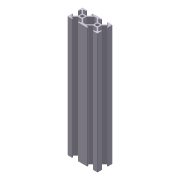
# Autodesk Inventor part: 8020-25-Double
Saved by Autodesk Inventor 2014 (Build 180170000, 170)
## iProperties
Created: 2014-08-06
Part Number: 8020-25-Double
Material: Generic
Document SubType Name: Modeling
Designer: Peele
Density: 1 g/cm^3
Appearance: Default
Author: Peele
Autodesk Inventor part; units mm, degrees
ref_plane "YZ Plane" through (0, 0, 0) normal (1, 0, 0) x (0, 1, 0)
ref_plane "XZ Plane" through (0, 0, 0) normal (0, 1, 0) x (-1, 0, 0)
ref_plane "XY Plane" through (0, 0, 0) normal (0, 0, 1) x (1, 0, 0)
sketch "Sketch1" plane through (0, 0, 0) normal (0, 0, 1) x (1, 0, 0)
  line L0 (-4.38, -4.38) -> (4.38, -4.38)
  line L1 (4.38, -4.38) -> (4.38, 4.38)
  line L2 (4.38, 4.38) -> (-4.38, 4.38)
  line L3 (-4.38, 4.38) -> (-4.38, -4.38)
  line L4 (-4.38, -4.38) -> (4.38, 4.38) construction
  line L5 (4.38, -4.38) -> (-4.38, 4.38) construction
  circle A0 centre (0, 0) radius 2.5
  dimension "d0" = 8.76
  dimension "d1" = 5
  constraints: 12 end point, 2 midpoint, 2 parallel, 2 perpendicular, 1 centre point, 1 coincident, 1 horizontal
  measures "d0" distance of L1.end L2.end
  measures "d1" diameter of A0
extrude "Extrusion1" add sketch "Sketch1" along normal mid plane 200
sketch "Sketch2" plane through (0, 0, 0) normal (0, 0, 1) x (1, 0, 0)
  line L0 (-4.38, 2.8668) -> (-10.36, 8.8468)
  line L1 (-10.36, 8.8468) -> (-10.36, 4.4)
  line L2 (-10.36, 4.4) -> (-12.5, 4.4)
  line L3 (-12.5, 4.4) -> (-12.5, 12.5)
  line L4 (-12.5, 12.5) -> (-4.4, 12.5)
  line L5 (-4.4, 12.5) -> (-4.4, 10.36)
  line L6 (-4.4, 10.36) -> (-8.8468, 10.36)
  line L7 (-8.8468, 10.36) -> (-2.8668, 4.38)
  line L8 (-2.8668, 4.38) -> (-4.38, 2.8668)
  line L9 (-4.38, 4.38) -> (4.38, 4.38) projected
  line L10 (-4.38, -4.38) -> (-4.38, 4.38) projected
  point P0 (0, 0)
  dimension "d4" = 12.5
  dimension "d5" = 2.14
  dimension "d6" = 8.1
  dimension "d7" = 2.14
  constraints: 18 end point, 6 perpendicular, 4 equal length, 2 point on line, 1 parallel, 1 vertical
  measures "d4" distance from line of point (0, 0) L4
  measures "d5" distance between parallel lines of L4 L6
  measures "d6" distance of L3.end L4.end
  measures "d7" distance between parallel lines of L0 L7
extrude "Extrusion2" add sketch "Sketch2" along normal up to surface (200 mm away) from surface at -100 contours L0 L1 L2 L3 L4 L5 L6 L7 L9 L10
pattern_circular "Circular Pattern1" count 4 over 360 about axis through (0, 0, 0) along (0, 0, 1) of "Extrusion2"
mirror "Mirror1" about plane through (12.5, 4.4, 0) normal (1, 0, 0) of "Extrusion2", "Extrusion1", "Circular Pattern1"
sketch "Sketch3" plane through (0, 0, 100) normal (0, 0, 1) x (1, 0, 0)
  line L0 (14.64, 4.4) -> (10.36, 4.4)
  line L1 (10.36, 4.4) -> (10.36, 9.2296)
  line L2 (10.36, 9.2296) -> (14.64, 9.2296)
  line L3 (14.64, 9.2296) -> (14.64, 4.4)
  line L4 (14.64, -4.4) -> (10.36, -4.4)
  line L5 (10.36, -4.4) -> (10.36, -8.8468)
  line L6 (10.36, -8.8468) -> (14.64, -8.8468)
  line L7 (14.64, -8.8468) -> (14.64, -4.4)
  constraints: 16 end point, 4 parallel, 2 horizontal, 2 perpendicular
extrude "Extrusion3" cut sketch "Sketch3" against normal up to next
fillet "Fillet4" radius 1 28 edges at (-10.36, 4.4, 0) (-10.36, -4.4, 0) (-12.5, -4.4, 0) (-12.5, 4.4, 0) (-12.5, 12.5, 0) (-4.4, 12.5, 0) (-4.4, 10.36, 0) (-4.4, -10.36, 0) (-4.4, -12.5, 0) (-12.5, -12.5, 0) (29.4, -10.36, 0) (29.4, -12.5, 0) (29.4, 10.36, 0) (29.4, 12.5, 0) (37.5, -4.4, 0) (35.36, -4.4, 0) (37.5, 12.5, 0) (37.5, -12.5, 0) (37.5, 4.4, 0) (35.36, 4.4, 0) (20.6, 10.36, 0) (20.6, 12.5, 0) (20.6, -12.5, 0) (20.6, -10.36, 0) (4.4, -12.5, 0) (4.4, -10.36, 0) (4.4, 10.36, 0) (4.4, 12.5, 0)
fillet "Fillet5" radius 0.75 16 edges at (-8.8468, -10.36, 0) (-10.36, -8.8468, 0) (8.8468, -10.36, 0) (10.36, -8.8468, 0) (14.64, -8.8468, 0) (16.1532, -10.36, 0) (33.8468, -10.36, 0) (35.36, -8.8468, 0) (33.8468, 10.36, 0) (8.8468, 10.36, 0) (35.36, 8.8468, 0) (16.1532, 10.36, 0) (14.64, 8.8468, 0) (10.36, 8.8468, 0) (-8.8468, 10.36, 0) (-10.36, 8.8468, 0)
fillet "Fillet6" radius 0.75 18 edges at (-4.38, -2.8668, 0) (-4.38, 2.8668, 0) (2.8668, 4.38, 0) (-2.8668, 4.38, 0) (-2.8668, -4.38, 0) (2.8668, -4.38, 0) (4.38, -2.8668, 0) (4.38, 2.8668, 0) (29.38, 2.8668, 0) (29.38, -2.8668, 0) (27.8668, 4.38, 0) (22.1332, 4.38, 0) (20.62, 2.8668, 0) (20.62, -2.8668, 0) (27.8668, -4.38, 0) (22.1332, -4.38, 0) (14.64, 9.2296, 0) (10.36, 9.2296, 0)
fillet "Fillet7" radius 0.75 222 edges at (-12.2071, -12.2071, 100) (-12.5, -8.45, 100) (-12.2071, -4.6929, 100) (-11.43, -4.4, 100) (-10.6529, -4.6929, 100) (-10.36, -6.2181, 100) (-9.897, -7.729, 100) (-6.8397, -5.3265, 100) (-4.4371, -2.8431, 100) (-4.38, 0, 100) (-4.4371, 2.8431, 100) (-6.8397, 5.3265, 100) (-9.897, 7.729, 100) (-10.36, 6.2181, 100) (-10.6529, 4.6929, 100) (-11.43, 4.4, 100) (-12.2071, 4.6929, 100) (-12.5, 8.45, 100) (-12.2071, 12.2071, 100) (-8.45, 12.5, 100) (-4.6929, 12.2071, 100) (-4.4, 11.43, 100) (-4.6929, 10.6529, 100) (-6.2181, 10.36, 100) (-7.729, 9.897, 100) (-5.3265, 6.8397, 100) (-2.8431, 4.4371, 100) (0, 4.38, 100) (2.8431, 4.4371, 100) (5.3265, 6.8397, 100) (7.729, 9.897, 100) (6.2181, 10.36, 100) (4.6929, 10.6529, 100) (4.4, 11.43, 100) (4.6929, 12.2071, 100) (12.5, 12.5, 100) (20.3071, 12.2071, 100) (20.6, 11.43, 100) (20.3071, 10.6529, 100) (18.7819, 10.36, 100) (17.271, 9.897, 100) (19.6735, 6.8397, 100) (22.1569, 4.4371, 100) (25, 4.38, 100) (27.8431, 4.4371, 100) (30.3265, 6.8397, 100) (32.729, 9.897, 100) (31.2181, 10.36, 100) (29.6929, 10.6529, 100) (29.4, 11.43, 100) (29.6929, 12.2071, 100) (33.45, 12.5, 100) (37.2071, 12.2071, 100) (37.5, 8.45, 100) (37.2071, 4.6929, 100) (36.43, 4.4, 100) (35.6529, 4.6929, 100) (35.36, 6.2181, 100) (34.897, 7.729, 100) (31.8397, 5.3265, 100) (29.4371, 2.8431, 100) (29.38, 0, 100) (29.4371, -2.8431, 100) (31.8397, -5.3265, 100) (34.897, -7.729, 100) (35.36, -6.2181, 100) (35.6529, -4.6929, 100) (36.43, -4.4, 100) (37.2071, -4.6929, 100) (37.5, -8.45, 100) (37.2071, -12.2071, 100) (33.45, -12.5, 100) (29.6929, -12.2071, 100) (29.4, -11.43, 100) (29.6929, -10.6529, 100) (31.2181, -10.36, 100) (32.729, -9.897, 100) (30.3265, -6.8397, 100) (27.8431, -4.4371, 100) (25, -4.38, 100) (22.1569, -4.4371, 100) (19.6735, -6.8397, 100) (17.271, -9.897, 100) (18.7819, -10.36, 100) (20.3071, -10.6529, 100) (20.6, -11.43, 100) (20.3071, -12.2071, 100) (12.5, -12.5, 100) (4.6929, -12.2071, 100) (4.4, -11.43, 100) (4.6929, -10.6529, 100) (6.2181, -10.36, 100) (7.729, -9.897, 100) (5.3265, -6.8397, 100) (2.8431, -4.4371, 100) (0, -4.38, 100) (-2.8431, -4.4371, 100) (-5.3265, -6.8397, 100) (-7.729, -9.897, 100) (-6.2181, -10.36, 100) (4.4371, 2.8431, 100) (7.37, 5.8568, 100) (10.2173, 8.7173, 100) (10.5555, 9.1186, 100) (12.5, 9.2296, 100) (14.4445, 9.1186, 100) (14.7827, 8.7173, 100) (17.63, 5.8568, 100) (20.5629, 2.8431, 100) (20.62, 0, 100) (20.5629, -2.8431, 100) (17.63, -5.8568, 100) (14.6164, -8.7897, 100) (12.5, -8.8468, 100) (10.3836, -8.7897, 100) (7.37, -5.8568, 100) (4.4371, -2.8431, 100) (4.38, 0, 100) (-2.5, 0, 100) (27.5, 0, 100) (22.1569, 4.4371, -100) (19.6735, 6.8397, -100) (17.271, 9.897, -100) (18.7819, 10.36, -100) (20.3071, 10.6529, -100) (20.6, 11.43, -100) (20.3071, 12.2071, -100) (12.5, 12.5, -100) (4.6929, 12.2071, -100) (4.4, 11.43, -100) (4.6929, 10.6529, -100) (6.2181, 10.36, -100) (7.729, 9.897, -100) (5.3265, 6.8397, -100) (2.8431, 4.4371, -100) (0, 4.38, -100) (-2.8431, 4.4371, -100) (-5.3265, 6.8397, -100) (-7.729, 9.897, -100) (-6.2181, 10.36, -100) (-4.6929, 10.6529, -100) (-4.4, 11.43, -100) (-4.6929, 12.2071, -100) (-8.45, 12.5, -100) (-12.2071, 12.2071, -100) (-12.5, 8.45, -100) (-12.2071, 4.6929, -100) (-11.43, 4.4, -100) (-10.6529, 4.6929, -100) (-10.36, 6.2181, -100) (-9.897, 7.729, -100) (-6.8397, 5.3265, -100) (-4.4371, 2.8431, -100) (-4.38, 0, -100) (-4.4371, -2.8431, -100) (-6.8397, -5.3265, -100) (-9.897, -7.729, -100) (-10.36, -6.2181, -100) (-10.6529, -4.6929, -100) (-11.43, -4.4, -100) (-12.2071, -4.6929, -100) (-12.5, -8.45, -100) (-12.2071, -12.2071, -100) (-8.45, -12.5, -100) (-4.6929, -12.2071, -100) (-4.4, -11.43, -100) (-4.6929, -10.6529, -100) (-6.2181, -10.36, -100) (-7.729, -9.897, -100) (-5.3265, -6.8397, -100) (-2.8431, -4.4371, -100) (0, -4.38, -100) (2.8431, -4.4371, -100) (5.3265, -6.8397, -100) (7.729, -9.897, -100) (6.2181, -10.36, -100) (4.6929, -10.6529, -100) (4.4, -11.43, -100) (4.6929, -12.2071, -100) (12.5, -12.5, -100) (20.3071, -12.2071, -100) (20.6, -11.43, -100) (20.3071, -10.6529, -100) (18.7819, -10.36, -100) (17.271, -9.897, -100) (19.6735, -6.8397, -100) (22.1569, -4.4371, -100) (25, -4.38, -100) (27.8431, -4.4371, -100) (30.3265, -6.8397, -100) (32.729, -9.897, -100) (31.2181, -10.36, -100) (29.6929, -10.6529, -100) (29.4, -11.43, -100) (29.6929, -12.2071, -100) (33.45, -12.5, -100) (37.2071, -12.2071, -100) (37.5, -8.45, -100) (37.2071, -4.6929, -100) (36.43, -4.4, -100) (35.6529, -4.6929, -100) (35.36, -6.2181, -100) (34.897, -7.729, -100) (31.8397, -5.3265, -100) (29.4371, -2.8431, -100) (29.38, 0, -100) (29.4371, 2.8431, -100) (31.8397, 5.3265, -100) (34.897, 7.729, -100) (35.36, 6.2181, -100) (35.6529, 4.6929, -100) (36.43, 4.4, -100) (37.2071, 4.6929, -100) (37.5, 8.45, -100) (37.2071, 12.2071, -100) (33.45, 12.5, -100) (29.6929, 12.2071, -100) (29.4, 11.43, -100) (29.6929, 10.6529, -100) (31.2181, 10.36, -100) (27.5, 0, -100) (-2.5, 0, -100)
fillet "Fillet8" radius 0.75 18 edges at (20.5629, -2.8431, -100) (17.63, -5.8568, -100) (14.6164, -8.7897, -100) (12.5, -8.8468, -100) (10.3836, -8.7897, -100) (7.37, -5.8568, -100) (4.4371, -2.8431, -100) (4.38, 0, -100) (4.4371, 2.8431, -100) (7.37, 5.8568, -100) (10.2173, 8.7173, -100) (10.5555, 9.1186, -100) (12.5, 9.2296, -100) (14.4445, 9.1186, -100) (14.7827, 8.7173, -100) (17.63, 5.8568, -100) (20.5629, 2.8431, -100) (20.62, 0, -100)
equation "\"d7\" = d5"
body "Solid1"
